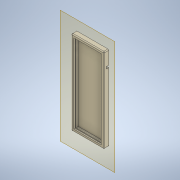
# Autodesk Inventor part: Case Parts
Saved by Autodesk Inventor 2022 (Build 260153000, 153)
## iProperties
Created: 2022-03-03
Part Number: Case Parts
Material: Generic
Document SubType Name: Modeling
Designer: Nathan Griffith
Density: 1 g/cm^3
Appearance: Default
Author: Nathan Griffith
Autodesk Inventor part; units mm, degrees
ref_plane "YZ Plane" through (0, 0, 0) normal (1, 0, 0) x (0, 1, 0)
ref_plane "XZ Plane" through (0, 0, 0) normal (0, 1, 0) x (-1, 0, 0)
ref_plane "XY Plane" through (0, 0, 0) normal (0, 0, 1) x (1, 0, 0)
ref_plane "Work Plane1" through (0, 0, 0) normal (0, 0, 1) x (1, 0, 0)
sketch "Sketch3" plane through (0, 0, 0) normal (0, 0, 1) x (1, 0, 0)
  line L0 (-60.325, -155.575) -> (60.325, -155.575)
  line L1 (60.325, -155.575) -> (60.325, 155.575)
  line L2 (60.325, 155.575) -> (-60.325, 155.575)
  line L3 (-60.325, 155.575) -> (-60.325, -155.575)
  line L4 (-60.325, -155.575) -> (60.325, 155.575) construction
  line L5 (60.325, -155.575) -> (-60.325, 155.575) construction
  point P0 (0, 0)
  dimension "d4" = 120.65
  dimension "d5" = 311.15
  constraints: 12 end point, 2 midpoint, 2 parallel, 1 horizontal, 1 perpendicular
  measures "d4" distance of L2.end L1.end
  measures "d5" distance of L1.end L0.end
extrude "Extrusion2" add sketch "Sketch3" against normal blind 18
sketch "Sketch4" plane through (0, 0, 0) normal (0, 0, 1) x (1, 0, 0)
  line L0 (-50.8, -146.05) -> (50.8, -146.05)
  line L1 (50.8, -146.05) -> (50.8, 146.05)
  line L2 (50.8, 146.05) -> (-50.8, 146.05)
  line L3 (-50.8, 146.05) -> (-50.8, -146.05)
  line L4 (-50.8, -146.05) -> (50.8, 146.05) construction
  line L5 (50.8, -146.05) -> (-50.8, 146.05) construction
  point P0 (0, 0)
  dimension "d8" = 101.6
  dimension "d9" = 292.1
  constraints: 12 end point, 2 midpoint, 2 parallel, 1 horizontal, 1 perpendicular
  measures "d8" distance of L2.end L1.end
  measures "d9" distance of L1.end L0.end
extrude "Extrusion3" cut sketch "Sketch4" against normal blind 5
sketch "Sketch5" plane through (0, 0, -5) normal (0, 0, 1) x (1, 0, 0)
  line L0 (50.8, 146.05) -> (50.8, -146.05) projected
  line L1 (-50.8, 146.05) -> (50.8, 146.05) projected
  line L2 (-50.8, -146.05) -> (-50.8, 146.05) projected
  line L3 (50.8, -146.05) -> (-50.8, -146.05) projected
  line L4 (47.8, -143.05) -> (47.8, 143.05)
  line L5 (47.8, 143.05) -> (-47.8, 143.05)
  line L6 (-47.8, 143.05) -> (-47.8, -143.05)
  line L7 (-47.8, -143.05) -> (47.8, -143.05)
  point P0 (0, 0)
  dimension "d12" = 3
  constraints: 8 end point, 3 other
  measures "d12" distance between parallel lines of L0 L4
extrude "Extrusion4" cut sketch "Sketch5" against normal blind 9 contours L7 L6 L5 L4
sketch "Sketch6" plane through (0, 0, -14) normal (0, 0, 1) x (1, 0, 0)
  line L0 (47.8, 143.05) -> (47.8, -143.05) projected
  line L1 (47.8, 143.05) -> (47.8, -143.05) projected
  line L2 (47.8, 104.95) -> (37.64, 104.95)
  line L3 (37.64, 104.95) -> (37.64, 97.33)
  line L4 (37.64, 97.33) -> (47.8, 97.33)
  line L5 (47.8, 97.33) -> (47.8, 104.95)
  line L6 (-47.8, 143.05) -> (47.8, 143.05) projected
  line L7 (47.8, 97.33) -> (60.325, 97.33)
  line L8 (60.325, 155.575) -> (60.325, -155.575) projected
  line L9 (60.325, 104.95) -> (47.8, 104.95)
  point P0 (0, 0)
  dimension "d16" = 10.16
  dimension "d17" = 7.62
  dimension "d18" = 38.1
  constraints: 12 end point, 3 point on line, 2 horizontal, 2 parallel, 2 perpendicular
  measures "d16" distance of L4.end L3.end
  measures "d17" distance of L3.end L2.end
  measures "d18" distance between parallel lines of L6 L2
extrude "Extrusion5" cut sketch "Sketch6" along normal mid plane 10.16
fillet "Fillet1" radius 3.175 8 edges at (0, 155.575, 0) (60.325, 0, 0) (0, -155.575, 0) (-60.325, 0, 0) (-60.325, 155.575, -9) (-60.325, -155.575, -9) (60.325, -155.575, -9) (60.325, 155.575, -9)
body "Solid2"
